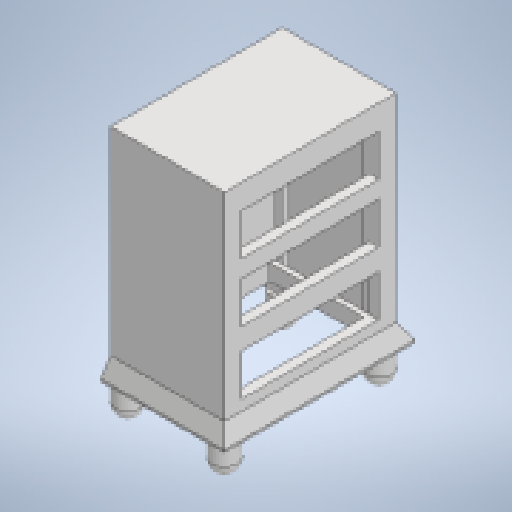
# Autodesk Inventor part: Comoda
Saved by Autodesk Inventor 2024 (Build 280153000, 153)
## iProperties
Created: 2025-02-23
Part Number: Comoda
Material: Genérico
Document SubType Name: Modeling
Designer: sergi
Density: 1 g/cm^3
Appearance: Valor por defecto
Author: sergi
Autodesk Inventor part; units mm, degrees
ref_plane "YZ Plane" through (0, 0, 0) normal (1, 0, 0) x (0, 1, 0)
ref_plane "XZ Plane" through (0, 0, 0) normal (0, 1, 0) x (-1, 0, 0)
ref_plane "XY Plane" through (0, 0, 0) normal (0, 0, 1) x (1, 0, 0)
sketch "Boceto1" plane through (0, 0, 0) normal (0, 1, 0) x (-1, 0, 0)
  line L0 (-148.5, 224) -> (148.5, 224)
  line L1 (148.5, 224) -> (148.5, -224)
  line L2 (148.5, -224) -> (-148.5, -224)
  line L3 (-148.5, -224) -> (-148.5, 224)
  line L4 (-148.5, 224) -> (148.5, -224) construction
  line L5 (148.5, 224) -> (-148.5, -224) construction
  point P0 (0, 0)
  dimension "d0" = 297
  dimension "d1" = 448
  constraints: 12 end point, 2 midpoint, 2 parallel, 1 horizontal, 1 perpendicular
  measures "d0" distance of L1.end L2.end
  measures "d1" distance of L0.end L1.end
extrude "Extrusión1" add sketch "Boceto1" along normal blind 564
sketch "Boceto2" plane through (0, 0, 0) normal (0, -1, 0) x (1, 0, 0)
  line L0 (148.5, -224) -> (-148.5, -224) projected
  line L1 (148.5, 224) -> (148.5, -224) projected
  line L2 (-148.5, 224) -> (148.5, 224) projected
  line L3 (-148.5, -224) -> (-148.5, 224) projected
  line L4 (-148.5, -224) -> (-148.5, 224) projected
  line L5 (-148.5, 224) -> (-104.5, 224)
  line L6 (-104.5, 224) -> (-104.5, 180)
  line L7 (-104.5, 180) -> (-148.5, 180)
  line L8 (-148.5, 180) -> (-148.5, 224)
  line L9 (148.5, 224) -> (104.5, 224)
  line L10 (104.5, 224) -> (104.5, 180)
  line L11 (104.5, 180) -> (148.5, 180)
  line L12 (148.5, 180) -> (148.5, 224)
  line L13 (148.5, -224) -> (104.5, -224)
  line L14 (104.5, -224) -> (104.5, -180)
  line L15 (104.5, -180) -> (148.5, -180)
  line L16 (148.5, -180) -> (148.5, -224)
  line L17 (-148.5, -224) -> (-104.5, -224)
  line L18 (-104.5, -224) -> (-104.5, -180)
  line L19 (-104.5, -180) -> (-148.5, -180)
  line L20 (-148.5, -180) -> (-148.5, -224)
  point P0 (0, 0)
  dimension "d4" = 44
  dimension "d5" = 44
  dimension "d6" = 44
  dimension "d7" = 44
  dimension "d8" = 44
  dimension "d9" = 44
  dimension "d10" = 44
  dimension "d11" = 44
  constraints: 32 end point, 8 parallel, 4 horizontal, 4 perpendicular
  measures "d4" distance of L6.end L7.end
  measures "d5" distance of L5.end L6.end
  measures "d6" distance of L11.end L10.end
  measures "d7" distance of L10.end L9.end
  measures "d8" distance of L14.end L15.end
  measures "d9" distance of L13.end L14.end
  measures "d10" distance of L19.end L18.end
  measures "d11" distance of L18.end L17.end
extrude "Extrusión2" cut sketch "Boceto2" against normal blind 28.5 contours L0 L18 L19 L3 L7 L6 L2 L10 L11 L1 L15 L14
sketch "Boceto3" plane through (0, 28.5, 0) normal (0, -1, 0) x (1, 0, 0)
  line L0 (-104.5, -224) -> (-104.5, -180) projected
  line L1 (104.5, -224) -> (-104.5, -224) projected
  line L2 (104.5, -180) -> (104.5, -224) projected
  line L3 (148.5, -180) -> (104.5, -180) projected
  line L4 (148.5, 180) -> (148.5, -180) projected
  line L5 (104.5, 180) -> (148.5, 180) projected
  line L6 (104.5, 224) -> (104.5, 180) projected
  line L7 (-104.5, 224) -> (104.5, 224) projected
  line L8 (-104.5, 180) -> (-104.5, 224) projected
  line L9 (-148.5, 180) -> (-104.5, 180) projected
  line L10 (-148.5, -180) -> (-148.5, 180) projected
  line L11 (-104.5, -180) -> (-148.5, -180) projected
  line L12 (148.5, 180) -> (123.5, 180)
  line L13 (123.5, 180) -> (123.5, -180)
  point P0 (0, 0)
  dimension "d14" = 25
  constraints: 4 end point, 2 point on line, 1 perpendicular
  measures "d14" distance of L4.start L12.end
extrude "Extrusión3" cut sketch "Boceto3" against normal blind 3 contours L0 L11 L10 L9 L8 L7 L6 L5 L13 L3 L2 L1
sketch "Boceto4" plane through (0, 0, 0) normal (0, -1, 0) x (1, 0, 0)
  line L0 (-104.5, 224) -> (104.5, 224) projected
  line L1 (-104.5, 224) -> (104.5, 224) projected
  line L2 (-104.5, 180) -> (-104.5, 224) projected
  line L3 (-148.5, 180) -> (-104.5, 180) projected
  line L4 (-148.5, -180) -> (-148.5, 180) projected
  line L5 (-104.5, -180) -> (-148.5, -180) projected
  line L6 (-104.5, -224) -> (-104.5, -180) projected
  line L7 (104.5, -224) -> (-104.5, -224) projected
  line L8 (104.5, -180) -> (104.5, -224) projected
  line L9 (123.5, -180) -> (104.5, -180) projected
  line L10 (123.5, 180) -> (123.5, -180) projected
  line L11 (104.5, 180) -> (123.5, 180) projected
  line L12 (104.5, 224) -> (104.5, 180) projected
  line L13 (104.5, 180) -> (148.5, 180) projected
  line L14 (148.5, 224) -> (148.5, 180) projected
  line L15 (104.5, 224) -> (148.5, 224) projected
  line L16 (104.5, 224) -> (104.5, 180) projected
  line L17 (123.5, 180) -> (123.5, -180) projected
  line L18 (148.5, -180) -> (123.5, -180) projected
  line L19 (148.5, 180) -> (148.5, -180) projected
  line L20 (123.5, 180) -> (148.5, 180) projected
  line L21 (148.5, -180) -> (104.5, -180) projected
  line L22 (104.5, -180) -> (104.5, -224) projected
  line L23 (148.5, -224) -> (104.5, -224) projected
  line L24 (148.5, -180) -> (148.5, -224) projected
  line L25 (-104.5, -224) -> (-104.5, -180) projected
  line L26 (-104.5, -180) -> (-148.5, -180) projected
  line L27 (-148.5, -224) -> (-148.5, -180) projected
  line L28 (-104.5, -224) -> (-148.5, -224) projected
  line L29 (-104.5, 180) -> (-104.5, 224) projected
  line L30 (-148.5, 224) -> (-104.5, 224) projected
  line L31 (-148.5, 180) -> (-148.5, 224) projected
  line L32 (-148.5, 180) -> (-104.5, 180) projected
  line L33 (-148.5, -224) -> (-148.5, -249)
  line L34 (-148.5, -249) -> (148.5, -249)
  line L35 (148.5, -249) -> (173.5, -249)
  line L36 (173.5, -249) -> (173.5, 224.4)
  line L37 (173.5, 224.4) -> (173.5, 249.4)
  line L38 (173.5, 249.4) -> (-148.5, 249.4)
  line L39 (-148.5, 249.4) -> (-148.5, -249)
  line L40 (-148.5, -249) -> (173.5, -249)
  line L41 (173.5, -249) -> (173.5, 249.4)
  point P0 (0, 0)
  dimension "d17" = 25
  dimension "d18" = 25
  dimension "d19" = 180
  dimension "d20" = 25
  dimension "d21" = 180
  constraints: 18 end point, 3 perpendicular, 2 collinear, 2 parallel, 1 horizontal, 1 vertical
  measures "d17" distance of L27.start L33.end
  measures "d18" distance of L34.end L35.end
  measures "d19" angle of L35 L34
  measures "d20" distance of L36.end L37.end
  measures "d21" angle of L37 L36
extrude "Extrusión4" add sketch "Boceto4" against normal blind 45.6 contours L30 L39 L38 L37 L36 L35 L34 L33 L28 L7 L23 L24 L19 L14 L15 L0
chamfer "Chaflán1" distance 25 distance2 40 3 edges at (173.5, 45.6, 0.2) (12.5, 45.6, 249.4) (12.5, 45.6, -249) measured on face at (12.5, 45.6, 248.9) measured on face at (173, 45.6, 0.2) measured on face at (12.5, 45.6, -248.5)
sketch "Boceto5" plane through (0, 31.5, 0) normal (0, -1, 0) x (1, 0, 0)
  line L0 (-104.5, 224) -> (104.5, 224) projected
  line L1 (-104.5, 180) -> (-104.5, 224) projected
  line L2 (-148.5, 180) -> (-104.5, 180) projected
  line L3 (-148.5, -180) -> (-148.5, 180) projected
  line L4 (-104.5, -180) -> (-148.5, -180) projected
  line L5 (-104.5, -224) -> (-104.5, -180) projected
  line L6 (104.5, -224) -> (-104.5, -224) projected
  line L7 (104.5, -180) -> (104.5, -224) projected
  line L8 (123.5, -180) -> (104.5, -180) projected
  line L9 (123.5, 180) -> (123.5, -180) projected
  line L10 (104.5, 180) -> (123.5, 180) projected
  line L11 (104.5, 224) -> (104.5, 180) projected
  line L12 (-148.5, 180) -> (-123.1, 180)
  line L13 (-123.1, 180) -> (-123.1, -180)
  line L14 (-104.5, 224) -> (-104.5, 198.6)
  line L15 (-104.5, 224) -> (-79.1, 224) construction
  line L16 (-104.5, 198.6) -> (104.5, 198.6)
  line L17 (104.5, -180) -> (104.5, -224) projected
  line L18 (104.5, -224) -> (104.5, -198.6)
  line L19 (104.5, -198.6) -> (-104.5, -198.6)
  point P0 (0, 0)
  dimension "d27" = 25.4
  dimension "d28" = 25.4
  dimension "d29" = 90
  dimension "d30" = 25.4
  constraints: 14 end point, 5 point on line, 4 perpendicular, 1 collinear, 1 horizontal
  measures "d27" distance of L2.start L12.end
  measures "d28" distance of L0.start L14.end
  measures "d29" angle of L14 L15
  measures "d30" distance of L6.start L18.end
extrude "Extrusión5" cut sketch "Boceto5" against normal blind 520 contours L16 L11 L10 L9 L8 L7 L19 L5 L4 L13 L2 L1
sketch "Boceto6" plane through (0, 0, 0) normal (0, -1, 0) x (1, 0, 0)
  line L0 (-104.5, 180) -> (-104.5, 224) projected
  line L1 (-104.5, 224) -> (104.5, 224) projected
  line L2 (104.5, 224) -> (104.5, 180) projected
  line L3 (104.5, 180) -> (148.5, 180) projected
  line L4 (148.5, 180) -> (148.5, -180) projected
  line L5 (148.5, -180) -> (104.5, -180) projected
  line L6 (104.5, -180) -> (104.5, -224) projected
  line L7 (104.5, -224) -> (-104.5, -224) projected
  line L8 (-104.5, -224) -> (-104.5, -180) projected
  line L9 (-104.5, -180) -> (-148.5, -180) projected
  line L10 (-148.5, -180) -> (-148.5, -249) projected
  line L11 (-148.5, -249) -> (173.5, -249) projected
  line L12 (173.5, -249) -> (173.5, 249.4) projected
  line L13 (173.5, 249.4) -> (-148.5, 249.4) projected
  line L14 (-148.5, 180) -> (-148.5, 249.4) projected
  line L15 (-148.5, 180) -> (-104.5, 180) projected
  line L16 (-148.5, -180) -> (-104.5, -224)
  circle A0 centre (-126.5, -202) radius 33
  line L17 (-104.5, 180) -> (-148.5, 224)
  line L18 (104.5, 224) -> (148.5, 180)
  line L19 (104.5, -224) -> (148.5, -180)
  circle A1 centre (126.5, 202) radius 33
  circle A2 centre (-126.5, 202) radius 33
  circle A3 centre (126.5, -202) radius 33
  point P0 (0, 0)
  dimension "d33" = 66
  dimension "d35" = 66
  dimension "d36" = 66
  dimension "d37" = 66
  constraints: 8 end point, 4 centre point, 4 midpoint, 2 point on line, 1 parallel, 1 perpendicular
  measures "d33" diameter of A0
  measures "d35" diameter of A1
  measures "d36" diameter of A2
  measures "d37" diameter of A3
extrude "Extrusión6" add sketch "Boceto6" along normal blind 90 contours L17 L14 A2 L1 L0 | L0 L1 A2 L14 L15 | L15 L14 L17 | A1 L4 L18 L1 | L1 L2 L3 L4 A1 | L18 L3 L2 | A3 L7 L19 L4 | L4 L5 L6 L7 A3 | L19 L6 L5 | A0 L10 L16 L7 | L7 L8 L9 L10 A0 | L16 L9 L8
fillet "Empalme1" radius 33 4 edges at (-159.5, -90, -202) (93.5, -90, -202) (93.5, -90, 202) (-159.5, -90, 202)
sketch "Boceto7" plane through (148.5, 564, 224) normal (1, 0, 0) x (0, 0, -1)
  line L0 (0, -518.4) -> (448, -518.4) projected
  line L1 (448, -518.4) -> (448, 0) projected
  line L2 (0, 0) -> (448, 0) projected
  line L3 (0, -518.4) -> (0, 0) projected
  line L4 (-0.4, -518.4) -> (-25.4, -558.4) projected
  line L5 (0, -518.4) -> (0, -490.25)
  line L6 (0, -490.25) -> (45, -490.25)
  line L7 (448, -518.4) -> (448, -490.25)
  line L8 (448, -490.25) -> (403, -490.25)
  line L9 (403, -490.25) -> (403, -381.75)
  line L10 (45, -490.25) -> (403, -490.25)
  line L11 (403, -490.25) -> (403, -381.75)
  line L12 (403, -381.75) -> (45, -381.75)
  line L13 (45, -381.75) -> (45, -490.25)
  line L14 (45, -381.75) -> (45, -371)
  line L15 (45, -371) -> (44, -326.1111)
  line L16 (44, -564) -> (44, -12.5) projected
  line L17 (44, -326.1111) -> (44, -217.6111)
  line L18 (44, -217.6111) -> (44, -172.7111)
  line L19 (404, -564) -> (404, -12.5) projected
  line L20 (44, -172.7111) -> (404, -172.7111)
  line L21 (404, -172.7111) -> (404, -64.2111)
  line L22 (404, -64.2111) -> (44, -64.2111)
  line L23 (44, -64.2111) -> (44, -172.7111)
  line L24 (44, -217.6111) -> (404, -217.6111)
  line L25 (404, -217.6111) -> (404, -326.1111)
  line L26 (404, -326.1111) -> (44, -326.1111)
  line L27 (44, -326.1111) -> (44, -217.6111)
  point P0 (224, -564)
  point P1 (44, -64.2111)
  dimension "d42" = 28.15
  dimension "d43" = 45
  dimension "d44" = 28.15
  dimension "d45" = 45
  dimension "d46" = 108.5
  dimension "d49" = 44.9
  dimension "d50" = 108.5
  dimension "d51" = 44.9
  dimension "d52" = 108.5
  constraints: 42 end point, 7 point on line, 6 parallel, 6 perpendicular, 3 horizontal
  measures "d42" distance of L0.start L5.end
  measures "d43" distance of L5.end L6.end
  measures "d44" distance of L0.end L7.end
  measures "d45" distance of L7.end L8.end
  measures "d46" distance of L8.end L9.end
  measures "d49" distance of L14.end L15.end
  measures "d50" distance of L15.end L17.end
  measures "d51" distance of L17.end L18.end
  measures "d52" distance of L21.end L20.end
extrude "Extrusión7" cut sketch "Boceto7" against normal up to surface (25 mm away) contours L13 L12 L9 L10 | L16 L24 L19 L26 | L16 L22 L19 L20
sketch "Boceto8" plane through (0, 31.5, 0) normal (0, -1, 0) x (1, 0, 0)
  line L0 (-123.1, -180) -> (-123.1, 180) projected
  line L1 (-148.5, 180) -> (-123.1, 180) projected
  line L2 (-148.5, -180) -> (-148.5, 180) projected
  line L3 (-123.1, -180) -> (-148.5, -180) projected
  line L4 (123.5, 180) -> (123.5, -180) projected
  line L5 (148.5, -180) -> (123.5, -180) projected
  line L6 (148.5, 180) -> (148.5, -180) projected
  line L7 (123.5, 180) -> (148.5, 180) projected
  line L8 (-123.1, 180) -> (123.5, 180)
  line L9 (123.5, 180) -> (123.5, 165.8)
  line L10 (123.5, 165.8) -> (-123.1, 165.8)
  line L11 (-123.1, 165.8) -> (-123.1, 180)
  line L12 (-123.1, -180) -> (-148.5, -180) projected
  line L13 (-123.1, -180) -> (123.5, -180)
  line L14 (123.5, -180) -> (123.5, -165.8)
  line L15 (123.5, -165.8) -> (-123.1, -165.8)
  line L16 (-123.1, -165.8) -> (-123.1, -180)
  point P0 (0, 0)
  point P1 (-123.1, -165.8)
  point P2 (-123.1, 165.8)
  dimension "d53" = 14.2
  dimension "d54" = 14.2
  constraints: 16 end point, 4 parallel, 2 horizontal, 2 perpendicular, 2 point on line
  measures "d53" distance of L8.end L9.end
  measures "d54" distance of L14.end L13.end
extrude "Extrusión8" add sketch "Boceto8" against normal up to surface (42.25 mm away) contours L0 L15 L4 L13 | L0 L8 L4 L10
